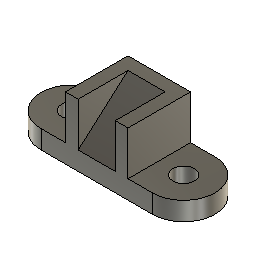
A2 v1 (Autodesk Fusion 360 design; units mm, degrees)
Autodesk Fusion 360 part; units mm, degrees
sketch "Sketch1" plane through (0, 0, 0) normal (0, 0, 1) x (1, 0, 0)
  line L0 (89, 32) -> (-89, 32)
  line L1 (-89, 32) -> (-89, -32)
  line L2 (-89, -32) -> (89, -32)
  line L3 (89, -32) -> (89, 32)
  line L4 (89, 32) -> (-89, -32) construction
  line L5 (-89, 32) -> (89, -32) construction
  circle A0 centre (-57, 0) radius 11
  circle A1 centre (57, 0) radius 11
  dimension "d1" = 178
  dimension "d2" = 64
  dimension "d13" = 22
  dimension "d14" = 22
  dimension "d21" = 114
  constraint horizontal L0
  constraint perpendicular L0 L1
  constraint parallel L0 L2
  constraint parallel L1 L3
  constraint coincident L4 origin
  constraint coincident L5 origin
  measures "d1" distance of L1.end L2.end
  measures "d2" distance of L0.end L1.end
  measures "d13" diameter of A0
  measures "d14" diameter of A1
  measures "d21" distance of A0.centre A1.centre
extrude "Extrude2" add sketch "Sketch1" along normal blind 19
fillet "Fillet3" radius 32 2 edges at (-89, -32, 9.5) (-89, 32, 9.5)
fillet "Fillet4" radius 32 2 edges at (89, -32, 9.5) (89, 32, 9.5)
sketch "Sketch2" plane through (0, 0, 19) normal (0, 0, 1) x (-1, 0, 0)
  arc A0 (-57, 32) -> (-57, -32) centre (-57, 0) ccw
  line L0 (-57, -32) -> (57, -32)
  arc A1 (57, -32) -> (57, 32) centre (57, 0) ccw
  line L1 (57, 32) -> (-57, 32)
  circle A2 centre (-57, 0) radius 11
  circle A3 centre (57, 0) radius 11
  line L2 (0, -32) -> (32, -32)
  line L3 (0, -32) -> (-32, -32)
  line L4 (32, -32) -> (32, 32)
  line L5 (-32, -32) -> (-32, 32)
  line L6 (32, 32) -> (19, 32)
  line L7 (-32, 32) -> (-19, 32)
  line L8 (19, 32) -> (19, -19)
  line L9 (-19, 32) -> (-19, -19)
  line L10 (19, -19) -> (-19, -19)
  dimension "d22" = 32
  dimension "d23" = 32
  dimension "d28" = 13
  dimension "d29" = 13
  dimension "d30" = 51
  dimension "d31" = 51
  constraint midpoint L0 L2.start
  constraint parallel L0 L3
  constraint coincident L1 L4.end
  constraint perpendicular L1 L4
  constraint coincident L1 L5.end
  constraint perpendicular L1 L5
  constraint perpendicular L4 L6
  constraint perpendicular L5 L7
  constraint perpendicular L1 L8
  constraint perpendicular L1 L9
  measures "d22" distance of L2.start L2.end
  measures "d23" distance of L2.start L3.end
  measures "d28" distance of L4.end L6.end
  measures "d29" distance of L5.end L7.end
  measures "d30" distance of L6.end L8.end
  measures "d31" distance of L7.end L9.end
extrude "Extrude3" add sketch "Sketch2" along normal blind 45 contours L0 L1 L2 L3 L4 L5 L6 L7 L8 L9 L10
sketch "Sketch3" plane through (19, 0, 0) normal (-1, 0, 0) x (0, -1, 0)
  line L0 (-19, 19) -> (32, 19)
  line L1 (32, 19) -> (32, 64)
  line L2 (32, 64) -> (-19, 64)
  line L3 (-19, 64) -> (-19, 19)
sketch "Sketch4" plane through (0, 0, 0) normal (1, 0, 0) x (0, 1, 0)
  line L0 (19, 19) -> (-32, 19)
  line L1 (19, 19) -> (19, 64)
  line L2 (19, 64) -> (-32, 19)
  dimension "d34" = 51
  dimension "d35" = 45
  constraint horizontal L0
  constraint perpendicular L0 L1
  measures "d34" distance of L0.start L0.end
  measures "d35" distance of L0.start L1.end
extrude "Extrude4" add sketch "Sketch4" along normal mid plane 38
equation "d32 = 64 mm - 19 mm"
